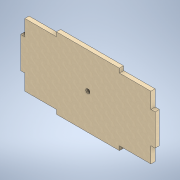
# Autodesk Inventor part: Platte4
Saved by Autodesk Inventor 2020.3 (Build 243373000, 373)
## iProperties
Created: 2020-11-28
Part Number: Platte4
Material: Generisch
Document SubType Name: Modeling
Designer: Stefan
Density: 1 g/cm^3
Appearance: Pappel
Author: Stefan
Autodesk Inventor part; units mm, degrees
ref_plane "YZ Plane" through (0, 0, 0) normal (1, 0, 0) x (0, 1, 0)
ref_plane "XZ Plane" through (0, 0, 0) normal (0, 1, 0) x (-1, 0, 0)
ref_plane "XY Plane" through (0, 0, 0) normal (0, 0, 1) x (1, 0, 0)
sketch "Skizze1" plane through (0, 0, 0) normal (0, 0, 1) x (1, 0, 0)
  line L0 (-150, -37.5) -> (-160, -37.5)
  line L1 (-160, -37.5) -> (-160, 37.5)
  line L2 (-160, 37.5) -> (-150, 37.5)
  line L3 (75, 75) -> (75, 85)
  line L4 (75, 85) -> (-75, 85)
  line L5 (-75, 85) -> (-75, 75)
  line L6 (0, -75) -> (0, 75) construction
  line L7 (-150, 0) -> (150, 0) construction
  line L8 (150, -37.5) -> (160, -37.5)
  line L9 (160, -37.5) -> (160, 37.5)
  line L10 (160, 37.5) -> (150, 37.5)
  line L11 (75, -75) -> (75, -85)
  line L12 (75, -85) -> (-75, -85)
  line L13 (-75, -85) -> (-75, -75)
  line L14 (-150, 75) -> (-150, 37.5)
  line L15 (-150, -37.5) -> (-150, -75)
  line L16 (-150, -75) -> (-75, -75)
  line L17 (75, -75) -> (150, -75)
  line L18 (150, -75) -> (150, -37.5)
  line L19 (150, 37.5) -> (150, 75)
  line L20 (150, 75) -> (75, 75)
  line L21 (-75, 75) -> (-150, 75)
  circle A0 centre (0, 0) radius 5
  dimension "d14" = 300
  dimension "d15" = 150
  dimension "d16" = 75
  dimension "d17" = 150
  dimension "d18" = 10
  dimension "d21" = 10
  dimension "d24" = 320
  dimension "d25" = 10
  dimension "d26" = 10
  constraints: 44 end point, 10 parallel, 8 symmetric about line, 5 perpendicular, 3 horizontal, 2 point on line, 1 centre point, 1 coincident
  measures "d14" distance of L14.start L19.end
  measures "d15" distance of L14.start L16.start
  measures "d16" distance of L0.end L1.end
  measures "d17" distance of L4.end L4.start
  measures "d18" distance of L1.end L2.end
  measures "d21" diameter of A0
  measures "d24" distance between parallel lines of L9 L1
  measures "d25" distance of L11.start L12.start
  measures "d26" distance of L10.start L19.start
extrude "Extrusion3" add sketch "Skizze1" along normal blind 10
equation "\"d9\" = d10"
equation "\"d10\" = 12"
